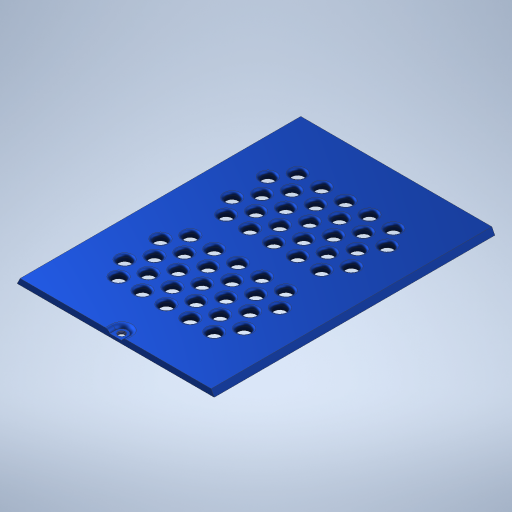
# Autodesk Inventor part: 12-5-Resized
Saved by Autodesk Inventor 2023 (Build 270158000, 158)
## iProperties
Created: 2024-02-28
Part Number: 12-5-Resized
Material: Generic
Document SubType Name: Modeling
Designer: ongyu
Density: 1 g/cm^3
Appearance: Default
Author: ongyu
Autodesk Inventor part; units mm, degrees
ref_plane "YZ Plane" through (0, 0, 0) normal (1, 0, 0) x (0, 1, 0)
ref_plane "XZ Plane" through (0, 0, 0) normal (0, 1, 0) x (-1, 0, 0)
ref_plane "XY Plane" through (0, 0, 0) normal (0, 0, 1) x (1, 0, 0)
sketch "Sketch1" plane through (0, 0, 0) normal (0, 0, 1) x (1, 0, 0)
  line L0 (-41.25, -1.25) -> (41.25, -1.25)
  line L1 (-40, 1.25) -> (40, 1.25)
  line L2 (0, 1.75) -> (0, -1.75) projected
  line L3 (-57.75, 0) -> (57.75, 0) projected
  line L4 (-40, 1.25) -> (-41.25, -1.25)
  line L5 (40, 1.25) -> (41.25, -1.25)
  line L6 (-40.4428, 0.3644) -> (40.4428, 0.3644) construction
  line L7 (0, -1.25) -> (0, 0.25)
  line L8 (0, 0.25) -> (40.5, 0.25)
  line L9 (40.5, 0.25) -> (-40.5, 0.25)
  point P0 (0, 0)
  dimension "d1" = 82.5
  dimension "d2" = 80
  dimension "d3" = 40
  dimension "d4" = 41.25
  dimension "d5" = 2.5
  dimension "d6" = 1.25
  dimension "d56" = 1.5
  dimension "d57" = 90
  dimension "d58" = 0
  constraints: 16 end point, 5 point on line, 3 horizontal, 1 midpoint
  measures "d1" distance of L0.start L0.end
  measures "d2" distance of L1.start L1.end
  measures "d3" distance from line of L1.start L2
  measures "d4" distance from line of L2 L0.start
  measures "d5" distance between parallel lines of L0 L1
  measures "d6" distance between parallel lines of L3 L1
  measures "d56" distance of L7.start L7.end
  measures "d57" angle of L7 L8
  measures "d58" distance between parallel lines of L9 L8
extrude "Extrusion1" add sketch "Sketch1" along normal blind 117.483
sketch "Sketch2" plane through (-40, 1.25, 0) normal (0, 1, 0) x (1, 0, 0)
  circle A0 centre (40, -114.983) radius 1.5
  line L0 (80, -117.483) -> (0, -117.483) projected
  circle A1 centre (40, -114.983) radius 2.5
  line L1 (42.5, -114.983) -> (42.5, -117.483)
  line L2 (37.5, -114.983) -> (37.5, -117.483)
  line L3 (0, 0) -> (0, -117.483) projected
  line L4 (80, 0) -> (80, -117.483) projected
  point P0 (40, 0)
  point P1 (40, -117.483)
  dimension "d9" = 3
  dimension "d10" = 2.5
  dimension "d13" = 5
  dimension "d59" = 40
  dimension "d61" = 80
  constraints: 4 end point, 2 centre point, 2 coincident, 2 perpendicular, 2 point on circle, 2 point on line, 1 tangent
  measures "d9" diameter of A0
  measures "d10" distance from line of L0 A0.centre
  measures "d13" diameter of A1
  measures "d59" distance from line of L3 A0.centre
  measures "d61" distance between parallel lines of L4 L3
extrude "Extrusion2" cut sketch "Sketch2" against normal through all contours A0
extrude "Extrusion3" cut sketch "Sketch2" against normal blind 1.25
sketch "Sketch3" plane through (-40, 1.25, 0) normal (0, 1, 0) x (1, 0, 0)
  point P0 (40, 0)
sketch "Sketch4" plane through (-40, 1.25, 0) normal (0, 1, 0) x (1, 0, 0)
  circle A0 centre (20, -21.25) radius 2.5
  line L0 (8.885, -21.25) -> (73.3803, -21.25)
  line L1 (80, 0) -> (0, 0) projected
  circle A1 centre (30, -21.25) radius 2.5
  circle A2 centre (40, -21.25) radius 2.5
  circle A3 centre (50, -21.25) radius 2.5
  circle A4 centre (60, -21.25) radius 2.5
  line L2 (5.7498, -28.75) -> (75.9698, -28.75)
  circle A5 centre (15, -28.75) radius 2.5
  circle A6 centre (25, -28.75) radius 2.5
  circle A7 centre (35, -28.75) radius 2.5
  circle A8 centre (45, -28.75) radius 2.5
  circle A9 centre (55, -28.75) radius 2.5
  circle A10 centre (65, -28.75) radius 2.5
  line L3 (-1.25, 0) -> (-1.25, -117.483) projected
  line L4 (81.25, 0) -> (81.25, -117.483) projected
  line L5 (40, 0) -> (40, -60)
  line L6 (40, 0) -> (100, 0) construction
  circle A11 centre (20, -36.25) radius 2.5
  circle A12 centre (30, -36.25) radius 2.5
  circle A13 centre (40, -36.25) radius 2.5
  circle A14 centre (50, -36.25) radius 2.5
  circle A15 centre (60, -36.25) radius 2.5
  circle A16 centre (65, -43.75) radius 2.5
  circle A17 centre (55, -43.75) radius 2.5
  circle A18 centre (45, -43.75) radius 2.5
  circle A19 centre (35, -43.75) radius 2.5
  circle A20 centre (25, -43.75) radius 2.5
  circle A21 centre (15, -43.75) radius 2.5
  circle A22 centre (20, -51.25) radius 2.5
  circle A23 centre (30, -51.25) radius 2.5
  circle A24 centre (40, -51.25) radius 2.5
  circle A25 centre (50, -51.25) radius 2.5
  circle A26 centre (60, -51.25) radius 2.5
  circle A27 centre (65, -58.75) radius 2.5
  circle A28 centre (55, -58.75) radius 2.5
  circle A29 centre (45, -58.75) radius 2.5
  circle A30 centre (35, -58.75) radius 2.5
  circle A31 centre (25, -58.75) radius 2.5
  circle A32 centre (15, -58.75) radius 2.5
  circle A33 centre (20, -66.25) radius 2.5
  circle A34 centre (30, -66.25) radius 2.5
  circle A35 centre (40, -66.25) radius 2.5
  circle A36 centre (50, -66.25) radius 2.5
  circle A37 centre (60, -66.25) radius 2.5
  circle A38 centre (65, -73.75) radius 2.5
  circle A39 centre (55, -73.75) radius 2.5
  circle A40 centre (45, -73.75) radius 2.5
  circle A41 centre (35, -73.75) radius 2.5
  circle A42 centre (25, -73.75) radius 2.5
  circle A43 centre (15, -73.75) radius 2.5
  circle A44 centre (20, -81.25) radius 2.5
  circle A45 centre (30, -81.25) radius 2.5
  circle A46 centre (40, -81.25) radius 2.5
  circle A47 centre (50, -81.25) radius 2.5
  circle A48 centre (60, -81.25) radius 2.5
  circle A49 centre (65, -88.75) radius 2.5
  circle A50 centre (55, -88.75) radius 2.5
  circle A51 centre (45, -88.75) radius 2.5
  circle A52 centre (35, -88.75) radius 2.5
  circle A53 centre (25, -88.75) radius 2.5
  circle A54 centre (15, -88.75) radius 2.5
  circle A55 centre (20, -96.25) radius 2.5
  circle A56 centre (30, -96.25) radius 2.5
  circle A57 centre (40, -96.25) radius 2.5
  circle A58 centre (50, -96.25) radius 2.5
  circle A59 centre (60, -96.25) radius 2.5
  circle A60 centre (65, -103.75) radius 2.5
  circle A61 centre (55, -103.75) radius 2.5
  circle A62 centre (45, -103.75) radius 2.5
  circle A63 centre (35, -103.75) radius 2.5
  circle A64 centre (25, -103.75) radius 2.5
  circle A65 centre (15, -103.75) radius 2.5
  line L7 (80, -117.483) -> (0, -117.483) projected
  dimension "d17" = 5
  dimension "d18" = 21.25
  dimension "d21" = 10
  dimension "d26" = 7.5
  dimension "d27" = 5
  dimension "d30" = 10
  dimension "d35" = 16.25
  dimension "d37" = 50
  dimension "d38" = 82.5
  dimension "d39" = 21.25
  dimension "d40" = 40
  dimension "d41" = 60
  dimension "d42" = 90
  dimension "d45" = 15
  dimension "d50" = 21.233
  constraints: 66 centre point, 8 end point, 5 horizontal, 2 point on line, 2 vertical, 1 perpendicular, 128 other
  measures "d17" diameter of A0
  measures "d18" distance between parallel lines of L0 L1
  measures "d21" distance of A0.centre A1.centre
  measures "d26" distance between parallel lines of L2 L0
  measures "d27" diameter of A5
  measures "d30" distance of A5.centre A6.centre
  measures "d35" distance from line of L3 A5.centre
  measures "d37" distance of A5.centre A10.centre
  measures "d38" distance between parallel lines of L4 L3
  measures "d39" distance from line of L3 A0.centre
  measures "d40" distance of A4.centre A0.centre
  measures "d41" distance of L5.start L5.end
  measures "d42" angle of L5 L6
  measures "d45" distance of A0.centre A11.centre
  measures "d50" distance from line of L7 A59.centre
extrude "Extrusion4" cut sketch "Sketch4" against normal up to surface (2.5 mm away) contours L0 A0 | A0 L0 | A1 L0 | L0 A1 | A2 L5 L0 | L0 L5 A2 | L5 A2 L0 | L0 A2 L5 | A3 L0 | L0 A3 | A4 L0 | L0 A4 | A5 L2 | L2 A5 | A6 L2 | L2 A6 | A7 L2 | L2 A7 | A8 L2 | L2 A8 | A9 L2 | L2 A9 | A10 L2 | L2 A10 | A13 L5 | L5 A13 | A24 L5 | L5 A24 | A11 | A12 | A14 | A15 | A16 | A17 | A18 | A19 | A20 | A21 | A22 | A23 | A25 | A26 | A33 | A34 | A35 | A36 | A37 | A38 | A39 | A40 | A41 | A42 | A43 | A44 | A45 | A46 | A47 | A48 | A49 | A50 | A51 | A52 | A53 | A54 | A55 | A56 | A57 | A58 | A59
fillet "Fillet2" radius 1 54 edges at (17.5, 1.25, 21.25) (22.5, 1.25, 28.75) (7.5, 1.25, 21.25) (12.5, 1.25, 28.75) (-2.5, 1.25, 21.25) (-12.5, 1.25, 21.25) (-22.5, 1.25, 21.25) (-27.5, 1.25, 28.75) (-17.5, 1.25, 28.75) (-7.5, 1.25, 28.75) (2.5, 1.25, 28.75) (17.5, 1.25, 36.25) (22.5, 1.25, 43.75) (12.5, 1.25, 43.75) (7.5, 1.25, 36.25) (-2.5, 1.25, 36.25) (-12.5, 1.25, 36.25) (-22.5, 1.25, 36.25) (-17.5, 1.25, 43.75) (-27.5, 1.25, 43.75) (-7.5, 1.25, 43.75) (2.5, 1.25, 43.75) (-2.5, 1.25, 51.25) (7.5, 1.25, 51.25) (17.5, 1.25, 51.25) (17.5, 1.25, 66.25) (-12.5, 1.25, 51.25) (-22.5, 1.25, 51.25) (-12.5, 1.25, 66.25) (-2.5, 1.25, 66.25) (7.5, 1.25, 66.25) (-22.5, 1.25, 66.25) (-17.5, 1.25, 73.75) (-27.5, 1.25, 73.75) (-7.5, 1.25, 73.75) (2.5, 1.25, 73.75) (12.5, 1.25, 73.75) (22.5, 1.25, 73.75) (17.5, 1.25, 81.25) (7.5, 1.25, 81.25) (-2.5, 1.25, 81.25) (-12.5, 1.25, 81.25) (-22.5, 1.25, 81.25) (-27.5, 1.25, 88.75) (-17.5, 1.25, 88.75) (-7.5, 1.25, 88.75) (2.5, 1.25, 88.75) (12.5, 1.25, 88.75) (22.5, 1.25, 88.75) (17.5, 1.25, 96.25) (7.5, 1.25, 96.25) (-2.5, 1.25, 96.25) (-12.5, 1.25, 96.25) (-22.5, 1.25, 96.25)
fillet "Fillet3" radius 2 3 edges at (2.5, 1.25, 116.233) (-2.5, 1.25, 116.233) (0, 1.25, 112.483)
thread "Thread1" size "M3x0.5" class "6H" standard "ANSI Metric M Profile" length 9
equation "\"d3\" = 0.5 * d2"
equation "\"d4\" = 0.5 * d1"
equation "\"d6\" = 0.5 * d5"
equation "\"d59\" = 0.5 * d61"
equation "\"d27\" = d17"
equation "\"d35\" = -0.5 * d37 + 0.5 * d38 + 0 * d17"
equation "\"d39\" = -0.5 * d40 + 0.5 * d38 + 0 * d17"
body "Solid1"
